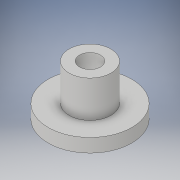
# Autodesk Inventor part: lower pin
Saved by Autodesk Inventor 2018 (Build 220112000, 112)
## iProperties
Created: 2021-03-17
Part Number: lower pin
Material: Generic
Document SubType Name: Modeling
Designer: Jyoti Soni
Density: 1 g/cm^3
Appearance: Default
Author: Jyoti Soni
Autodesk Inventor part; units mm, degrees
ref_plane "YZ Plane" through (0, 0, 0) normal (1, 0, 0) x (0, 1, 0)
ref_plane "XZ Plane" through (0, 0, 0) normal (0, 1, 0) x (-1, 0, 0)
ref_plane "XY Plane" through (0, 0, 0) normal (0, 0, 1) x (1, 0, 0)
sketch "Sketch1" plane through (0, 0, 0) normal (0, 0, 1) x (1, 0, 0)
  line L0 (0, 2.6898) -> (0, -4.5766) construction
  line L1 (1.25, -3.4484) -> (1.25, 2.5516)
  line L2 (1.25, 2.5516) -> (2.5, 2.5516)
  line L3 (2.5, 2.5516) -> (2.5, -1.8319)
  line L4 (2.5, -1.8319) -> (5, -1.8319)
  line L5 (5, -1.8319) -> (5, -3.4484)
  line L6 (5, -3.4484) -> (1.25, -3.4484)
  point P0 (0, 0)
  dimension "d0" = 1.25
  dimension "d1" = 6
  dimension "d2" = 5
  dimension "d3" = 1.25
  constraints: 14 end point, 5 perpendicular, 2 vertical
  measures "d0" distance between parallel lines of L0 L1
  measures "d1" distance of L1.start L1.end
  measures "d2" distance between parallel lines of L0 L5
  measures "d3" distance of L1.end L2.end
revolve "Revolution1" add sketch "Sketch1" angle 360 about axis through (0, 2.6898, 0) along (0, -1, 0)
body "Solid1"
